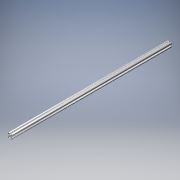
# Autodesk Inventor part: Aluminium extrusion profile 2020
Saved by Autodesk Inventor 2019.4 (Build 234330000, 330)
## iProperties
Part Number: Aluminium extrusion profile 2020
Material: Hliník 6061
Document SubType Name: Modeling
Designer: HP Genius
Density: 2.7 g/cm^3
Appearance: Hliník – plochý
Mass: 323.554 g
Surface Area: 1156.31 cm^2
Volume: 119.835 cm^3
Author: HP Genius
Autodesk Inventor part; units mm, degrees
ref_plane "YZ Plane" through (0, 0, 0) normal (1, 0, 0) x (0, 1, 0)
ref_plane "XZ Plane" through (0, 0, 0) normal (0, 1, 0) x (-1, 0, 0)
ref_plane "XY Plane" through (0, 0, 0) normal (0, 0, 1) x (1, 0, 0)
sketch "Náčrt1" plane through (0, 0, 0) normal (0, 1, 0) x (-1, 0, 0)
  circle A0 centre (10, 10) radius 2.5
  line L0 (20, 13) -> (20, 20)
  line L1 (20, 20) -> (13, 20)
  line L2 (7, 20) -> (0, 20)
  line L3 (0, 20) -> (0, 13)
  line L4 (7, 0) -> (0, 0)
  line L5 (0, 7) -> (0, 0)
  line L6 (0, 0) -> (7, 0)
  line L7 (18.2, 13) -> (20, 13)
  line L8 (13, 18.2) -> (13, 20)
  line L9 (7, 20) -> (7, 18.2)
  line L10 (0, 13) -> (1.8, 13)
  line L11 (1.8, 7) -> (0, 7)
  line L12 (7, 1.8) -> (7, 0)
  line L13 (1.8, 15.5002) -> (3.3002, 15.5002)
  line L14 (4.4112, 18.2) -> (4.4112, 16.7)
  line L15 (3.3002, 15.5002) -> (3.5002, 15.5002)
  line L16 (4.4112, 16.7) -> (4.4112, 16.5)
  line L17 (3.5002, 15.5002) -> (6.0002, 13.0002)
  line L18 (4.4112, 16.5) -> (6.9112, 14)
  line L19 (7, 18.2) -> (4.4112, 18.2)
  line L20 (1.8, 13) -> (1.8, 15.5002)
  line L21 (4.5002, 3.5002) -> (7.0002, 6.0002)
  line L22 (3.5002, 4.5002) -> (6.0002, 7.0002)
  line L23 (1.8, 4.5002) -> (3.5002, 4.5002)
  line L24 (4.5002, 1.8) -> (4.5002, 3.5002)
  line L25 (15.5002, 3.5002) -> (13.0002, 6.0002)
  line L26 (16.4498, 4.5506) -> (14.0002, 7.0002)
  line L27 (15.4112, 16.5) -> (12.9112, 14)
  line L28 (16.4114, 15.5002) -> (13.9112, 13)
  line L29 (12.9112, 14) -> (6.9112, 14)
  line L30 (6.0002, 13.0002) -> (6.0002, 7.0002)
  line L31 (7.0002, 6.0002) -> (13.0002, 6.0002)
  line L32 (14.0002, 7.0002) -> (13.9554, 13.0442)
  line L33 (15.4112, 16.5) -> (15.4112, 18.2)
  line L34 (16.4114, 15.5002) -> (18.2, 15.4679)
  line L35 (20, 7) -> (20, 0)
  line L36 (20, 0) -> (13, 0)
  line L37 (13, 0) -> (13, 1.8)
  line L38 (18.2, 7) -> (20, 7)
  line L39 (15.5002, 3.5002) -> (15.5002, 1.8)
  line L40 (16.4498, 4.5506) -> (18.2, 4.5506)
  line L41 (18.2, 7) -> (18.2, 4.5506)
  line L42 (15.5002, 1.8) -> (13, 1.8)
  line L43 (18.2, 13) -> (18.2, 15.4679)
  line L44 (15.4112, 18.2) -> (13, 18.2)
  line L45 (7, 1.8) -> (4.5002, 1.8)
  line L46 (1.8, 4.5002) -> (1.8, 7)
  line L47 (20, 20) -> (13, 20)
  line L48 (13, 20) -> (13, 18.2)
  line L49 (13, 18.2) -> (15.4112, 18.2)
  line L50 (15.4112, 18.2) -> (15.4112, 16.5)
  line L51 (12.9112, 14) -> (6.9112, 14)
  line L52 (6.9112, 14) -> (4.4112, 16.5)
  line L53 (4.4112, 16.5) -> (4.4112, 18.2)
  line L54 (4.4112, 18.2) -> (7, 18.2)
  line L55 (0, 20) -> (0, 20)
  line L56 (1.8, 13) -> (1.8, 15.5002)
  line L57 (1.8, 15.5002) -> (3.5002, 15.5002)
  line L58 (3.5002, 15.5002) -> (6.0002, 13.0002)
  line L59 (6.0002, 13.0002) -> (6.0002, 7.0002)
  line L60 (6.0002, 7.0002) -> (3.5002, 4.5002)
  line L61 (3.5002, 4.5002) -> (1.8, 4.5002)
  line L62 (1.8, 4.5002) -> (1.8, 7)
  line L63 (1.8, 7) -> (0, 7)
  line L64 (0, 7) -> (0, 0)
  line L65 (0, 0) -> (7, 0)
  line L66 (7, 0) -> (7, 1.8)
  line L67 (7, 1.8) -> (4.5002, 1.8)
  line L68 (4.5002, 1.8) -> (4.5002, 3.5002)
  line L69 (4.5002, 3.5002) -> (7.0002, 6.0002)
  line L70 (7.0002, 6.0002) -> (13.0002, 6.0002)
  line L71 (13.0002, 6.0002) -> (15.5002, 3.5002)
  line L72 (15.5002, 1.8) -> (13, 1.8)
  line L73 (13, 0) -> (20, 0)
  line L74 (20, 0) -> (20, 7)
  line L75 (20, 7) -> (18.2, 7)
  line L76 (7, 20) -> (0, 20)
  line L77 (0, 20) -> (0, 13)
  line L78 (0, 13) -> (1.8, 13)
  line L79 (1.8, 13) -> (1.8, 15.5002)
  line L80 (1.8, 15.5002) -> (3.5002, 15.5002)
  line L81 (6.0002, 13.0002) -> (6.0002, 7.0002)
  line L82 (6.0002, 7.0002) -> (3.5002, 4.5002)
  line L83 (1.8, 4.5002) -> (1.8, 7)
  line L84 (1.8, 7) -> (0, 7)
  line L85 (0, 7) -> (0, 0)
  line L86 (0, 0) -> (7, 0)
  line L87 (7, 0) -> (7, 1.8)
  line L88 (7, 1.8) -> (4.5002, 1.8)
  line L89 (4.5002, 1.8) -> (4.5002, 3.5002)
  line L90 (4.5002, 3.5002) -> (7.0002, 6.0002)
  line L91 (7.0002, 6.0002) -> (13.0002, 6.0002)
  line L92 (13.0002, 6.0002) -> (15.5002, 3.5002)
  line L93 (15.5002, 3.5002) -> (15.5002, 1.8)
  line L94 (15.5002, 1.8) -> (13, 1.8)
  line L95 (13, 1.8) -> (13, 0)
  line L96 (13, 0) -> (20, 0)
  line L97 (20, 0) -> (20, 7)
  line L98 (20, 7) -> (18.2, 7)
  line L99 (18.2, 7) -> (18.2, 4.5506)
  line L100 (18.2, 4.5506) -> (16.4498, 4.5506)
  line L101 (16.4498, 4.5506) -> (14.0002, 7.0002)
  line L102 (14.0002, 7.0002) -> (13.9554, 13.0442)
  line L103 (13.9554, 13.0442) -> (16.4114, 15.5002)
  line L104 (16.4114, 15.5002) -> (18.2, 15.4679)
  line L105 (18.2, 15.4679) -> (18.2, 13)
  line L106 (18.2, 13) -> (20, 13)
  line L107 (20, 13) -> (20, 20)
  line L108 (20, 20) -> (13, 20)
  line L109 (13, 20) -> (13, 18.2)
  line L110 (13, 18.2) -> (15.4112, 18.2)
  line L111 (15.4112, 18.2) -> (15.4112, 16.5)
  line L112 (15.4112, 16.5) -> (12.9112, 14)
  line L113 (12.9112, 14) -> (6.9112, 14)
  line L114 (6.9112, 14) -> (4.4112, 16.5)
  line L115 (4.4112, 16.5) -> (4.4112, 18.2)
  line L116 (4.4112, 18.2) -> (7, 18.2)
  line L117 (7, 18.2) -> (7, 20)
  dimension "d1" = 20
  dimension "d46" = 1.5
  dimension "d49" = 1.4142
  dimension "d53" = 1.4142
  dimension "d56" = 1.4142
  dimension "d60" = 1.8
  dimension "d61" = 1.8
  dimension "d62" = 1.8
  dimension "d63" = 1.8
  dimension "d65" = 1.8
  dimension "d66" = 1.8
  dimension "d67" = 1.8
  dimension "d72" = 2.5
  dimension "d73" = 7
  dimension "d74" = 7
  dimension "d75" = 7
  dimension "d76" = 7
  dimension "d77" = 7
  dimension "d78" = 7
  dimension "d79" = 7
  dimension "d80" = 7
  dimension "d81" = 20
  dimension "d82" = 5
  dimension "d86" = 10
  dimension "d87" = 10
  constraints: 236 end point, 43 collinear, 39 perpendicular, 8 parallel, 8 point on line, 7 horizontal, 5 vertical, 1 centre point
  measures "d1" distance of L0.end L2.end
  measures "d46" distance of L14.start L14.end
  measures "d49" distance between parallel lines of L21 L22
  measures "d53" distance between parallel lines of L25 L26
  measures "d56" distance between parallel lines of L28 L27
  measures "d60" distance of L8.start L1.end
  measures "d61" distance of L2.start L9.end
  measures "d62" distance of L11.start L5.start
  measures "d63" distance of L12.start L4.start
  measures "d65" distance of L7.start L0.start
  measures "d66" distance of L36.end L37.end
  measures "d67" distance of L38.start L38.end
  measures "d72" horizontal distance of L16.end L18.end
  measures "d73" distance of L2.end L3.end
  measures "d74" distance of L0.start L0.end
  measures "d75" distance of L35.end L38.end
  measures "d76" distance of L5.start L4.end
  measures "d77" distance of L2.start L2.end
  measures "d78" distance of L0.end L1.end
  measures "d79" distance of L35.end L36.end
  measures "d80" distance of L4.end L4.start
  measures "d81" distance of L4.end L2.end
  measures "d82" diameter of A0
  measures "d86" distance from line of L2 A0.centre
  measures "d87" distance from line of L5 A0.centre
extrude "Vysunutí1" add sketch "Náčrt1" along normal blind 750
fillet "Zaoblení1" radius 1.5 4 edges at (-20, 375, 20) (-20, 375, 0) (0, 375, 0) (0, 375, 20)
chamfer "Zkosení1" distance 1 angle 45 8 edges at (-13, 375, 20) (-7, 375, 20) (0, 375, 7) (0, 375, 13) (-20, 375, 13) (-20, 375, 7) (-7, 375, 0) (-13, 375, 0)
sketch "Sketch2" plane through (-6.9112, 0, 14) normal (0, 0, 1) x (1, 0, 0)
  circle A0 centre (-3.0888, 10) radius 2.75
  circle A1 centre (-3.0888, 40.5) radius 2.75
  circle A2 centre (-3.0888, 65.5) radius 2.75
  line L0 (6.9112, 0) -> (6.9112, 750) projected
  line L1 (-11.5888, 0) -> (-7.0888, 0) projected
  dimension "d88" = 5.5
  dimension "d89" = 5.5
  dimension "d90" = 5.5
  dimension "d91" = 10
  dimension "d92" = 10
  dimension "d93" = 10
  dimension "d94" = 25
  dimension "d95" = 10
  dimension "d96" = 25
  constraints: 3 centre point
  measures "d88" diameter of A0
  measures "d89" diameter of A1
  measures "d90" diameter of A2
  measures "d91" distance from line of L0 A1.centre
  measures "d92" distance from line of L0 A0.centre
  measures "d93" distance from line of L0 A2.centre
  measures "d94" distance of A1.centre A2.centre
  measures "d95" distance from line of L1 A0.centre
extrude "Extrusion2" cut sketch "Sketch2" against normal blind 10
